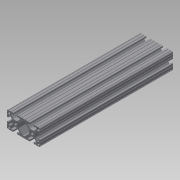
# Autodesk Inventor part: 1530-LITE
Saved by Autodesk Inventor 2013 (Build 170138000, 138)
## iProperties
Created: 2014-04-23
Part Number: 1530-LITE
Material: Generic
Document SubType Name: Modeling
Density: 1 g/cm^3
Vendor: 80/20 Inc.
Engineer: Ross Bowman
Designer: Ross Bowman
Catalog Web Link: 8020.net
Company: 80/20 Inc.
Author: Ross Bowman
Keywords: 80/20 , 8020 , T-Slot , Extrusion
Material: 6105-T5 Aluminum
Autodesk Inventor part; units mm, degrees
ref_plane "YZ Plane" through (0, 0, 0) normal (1, 0, 0) x (0, 1, 0)
ref_plane "XZ Plane" through (0, 0, 0) normal (0, 1, 0) x (-1, 0, 0)
ref_plane "XY Plane" through (0, 0, 0) normal (0, 0, 1) x (1, 0, 0)
sketch "Sketch1" plane through (0, 0, 0) normal (0, 0, 1) x (1, 0, 0)
  arc A0 (-31.2928, -17.2466) -> (-30.9118, -16.8656) centre (-31.2928, -16.8656) ccw
  line L0 (-33.5026, -17.2466) -> (-31.2928, -17.2466)
  arc A1 (-36.2966, -14.4526) -> (-33.5026, -17.2466) centre (-33.5026, -14.4526) ccw
  line L1 (-36.2966, -12.2428) -> (-36.2966, -14.4526)
  arc A2 (-35.9156, -11.8618) -> (-36.2966, -12.2428) centre (-35.9156, -12.2428) ccw
  line L2 (-31.2928, -11.8618) -> (-35.9156, -11.8618)
  arc A3 (-30.9118, -12.2428) -> (-31.2928, -11.8618) centre (-31.2928, -12.2428) ccw
  line L3 (-30.9118, -16.8656) -> (-30.9118, -12.2428)
  arc A4 (2.0655, 14.8293) -> (-2.0655, 14.8293) centre (0, 12.7638) ccw
  line L4 (10.9278, 5.9669) -> (2.0655, 14.8293)
  arc A5 (12.319, 2.6083) -> (10.9278, 5.9669) centre (7.5692, 2.6083) ccw
  line L5 (12.319, -2.6083) -> (12.319, 2.6083)
  arc A6 (10.9278, -5.9669) -> (12.319, -2.6083) centre (7.5692, -2.6083) ccw
  line L6 (2.0655, -14.8293) -> (10.9278, -5.9669)
  arc A7 (-2.0655, -14.8293) -> (2.0655, -14.8293) centre (0, -12.7638) ccw
  line L7 (-10.9278, -5.9669) -> (-2.0655, -14.8293)
  arc A8 (-12.319, -2.6083) -> (-10.9278, -5.9669) centre (-7.5692, -2.6083) ccw
  line L8 (-12.319, 2.6083) -> (-12.319, -2.6083)
  arc A9 (-10.9278, 5.9669) -> (-12.319, 2.6083) centre (-7.5692, 2.6083) ccw
  line L9 (-2.0655, 14.8293) -> (-10.9278, 5.9669)
  circle A10 centre (19.05, 0) radius 3.3274
  arc A11 (30.9118, -16.8656) -> (31.2928, -17.2466) centre (31.2928, -16.8656) ccw
  line L10 (30.9118, -12.2428) -> (30.9118, -16.8656)
  arc A12 (31.2928, -11.8618) -> (30.9118, -12.2428) centre (31.2928, -12.2428) ccw
  line L11 (35.9156, -11.8618) -> (31.2928, -11.8618)
  arc A13 (36.2966, -12.2428) -> (35.9156, -11.8618) centre (35.9156, -12.2428) ccw
  line L12 (36.2966, -14.4526) -> (36.2966, -12.2428)
  arc A14 (33.5026, -17.2466) -> (36.2966, -14.4526) centre (33.5026, -14.4526) ccw
  line L13 (31.2928, -17.2466) -> (33.5026, -17.2466)
  arc A15 (31.2928, 17.2466) -> (30.9118, 16.8656) centre (31.2928, 16.8656) ccw
  line L14 (33.5026, 17.2466) -> (31.2928, 17.2466)
  arc A16 (36.2966, 14.4526) -> (33.5026, 17.2466) centre (33.5026, 14.4526) ccw
  line L15 (36.2966, 12.2428) -> (36.2966, 14.4526)
  arc A17 (35.9156, 11.8618) -> (36.2966, 12.2428) centre (35.9156, 12.2428) ccw
  line L16 (31.2928, 11.8618) -> (35.9156, 11.8618)
  arc A18 (30.9118, 12.2428) -> (31.2928, 11.8618) centre (31.2928, 12.2428) ccw
  line L17 (30.9118, 16.8656) -> (30.9118, 12.2428)
  circle A19 centre (-19.05, 0) radius 3.3274
  arc A20 (-30.9118, 16.8656) -> (-31.2928, 17.2466) centre (-31.2928, 16.8656) ccw
  line L18 (-30.9118, 12.2428) -> (-30.9118, 16.8656)
  arc A21 (-31.2928, 11.8618) -> (-30.9118, 12.2428) centre (-31.2928, 12.2428) ccw
  line L19 (-35.9156, 11.8618) -> (-31.2928, 11.8618)
  arc A22 (-36.2966, 12.2428) -> (-35.9156, 11.8618) centre (-35.9156, 12.2428) ccw
  line L20 (-36.2966, 14.4526) -> (-36.2966, 12.2428)
  arc A23 (-33.5026, 17.2466) -> (-36.2966, 14.4526) centre (-33.5026, 14.4526) ccw
  line L21 (-31.2928, 17.2466) -> (-33.5026, 17.2466)
  arc A24 (-3.2004, -19.05) -> (-4.7244, -19.05) centre (-3.9624, -19.05) ccw
  line L22 (-3.2004, -19.05) -> (3.2004, -19.05)
  arc A25 (4.7244, -19.05) -> (3.2004, -19.05) centre (3.9624, -19.05) ccw
  line L23 (4.7244, -19.05) -> (9.5504, -19.05)
  arc A26 (11.0744, -19.05) -> (9.5504, -19.05) centre (10.3124, -19.05) ccw
  line L24 (11.0744, -19.05) -> (13.4112, -19.05)
  arc A27 (13.4112, -19.05) -> (14.986, -17.4752) centre (13.4112, -17.4752) ccw
  line L25 (14.986, -17.4752) -> (14.986, -16.5608)
  arc A28 (14.986, -16.5608) -> (13.4112, -14.986) centre (13.4112, -16.5608) ccw
  line L26 (13.4112, -14.986) -> (12.573, -14.986)
  arc A29 (12.573, -14.986) -> (12.192, -15.367) centre (12.573, -15.367) ccw
  line L27 (12.192, -15.367) -> (12.192, -15.4432)
  arc A30 (11.811, -15.8242) -> (12.192, -15.4432) centre (11.811, -15.4432) ccw
  line L28 (11.811, -15.8242) -> (10.033, -15.8242)
  arc A31 (8.763, -14.5542) -> (10.033, -15.8242) centre (10.033, -14.5542) ccw
  line L29 (8.763, -14.5542) -> (8.763, -12.9683)
  arc A32 (9.135, -12.0703) -> (8.763, -12.9683) centre (10.033, -12.9683) ccw
  line L30 (9.135, -12.0703) -> (13.0831, -8.1222)
  arc A33 (16.4417, -6.731) -> (13.0831, -8.1222) centre (16.4417, -11.4808) ccw
  line L31 (16.4417, -6.731) -> (21.6583, -6.731)
  arc A34 (25.0169, -8.1222) -> (21.6583, -6.731) centre (21.6583, -11.4808) ccw
  line L32 (25.0169, -8.1222) -> (28.965, -12.0703)
  arc A35 (29.337, -12.9683) -> (28.965, -12.0703) centre (28.067, -12.9683) ccw
  line L33 (29.337, -12.9683) -> (29.337, -14.5542)
  arc A36 (28.067, -15.8242) -> (29.337, -14.5542) centre (28.067, -14.5542) ccw
  line L34 (28.067, -15.8242) -> (26.289, -15.8242)
  arc A37 (25.908, -15.4432) -> (26.289, -15.8242) centre (26.289, -15.4432) ccw
  line L35 (25.908, -15.4432) -> (25.908, -15.367)
  arc A38 (25.908, -15.367) -> (25.527, -14.986) centre (25.527, -15.367) ccw
  line L36 (25.527, -14.986) -> (24.6888, -14.986)
  arc A39 (24.6888, -14.986) -> (23.114, -16.5608) centre (24.6888, -16.5608) ccw
  line L37 (23.114, -16.5608) -> (23.114, -17.4752)
  arc A40 (23.114, -17.4752) -> (24.6888, -19.05) centre (24.6888, -17.4752) ccw
  line L38 (24.6888, -19.05) -> (27.0256, -19.05)
  arc A41 (28.5496, -19.05) -> (27.0256, -19.05) centre (27.7876, -19.05) ccw
  line L39 (28.5496, -19.05) -> (33.3756, -19.05)
  arc A42 (34.8996, -19.05) -> (33.3756, -19.05) centre (34.1376, -19.05) ccw
  line L40 (34.8996, -19.05) -> (34.925, -19.05)
  arc A43 (34.925, -19.05) -> (38.1, -15.875) centre (34.925, -15.875) ccw
  line L41 (38.1, -15.875) -> (38.1, -15.8496)
  arc A44 (38.1, -14.3256) -> (38.1, -15.8496) centre (38.1, -15.0876) ccw
  line L42 (38.1, -14.3256) -> (38.1, -9.4996)
  arc A45 (38.1, -7.9756) -> (38.1, -9.4996) centre (38.1, -8.7376) ccw
  line L43 (38.1, -7.9756) -> (38.1, -5.6388)
  arc A46 (38.1, -5.6388) -> (36.5252, -4.064) centre (36.5252, -5.6388) ccw
  line L44 (36.5252, -4.064) -> (35.6108, -4.064)
  arc A47 (35.6108, -4.064) -> (34.036, -5.6388) centre (35.6108, -5.6388) ccw
  line L45 (34.036, -5.6388) -> (34.036, -6.477)
  arc A48 (34.036, -6.477) -> (34.417, -6.858) centre (34.417, -6.477) ccw
  line L46 (34.417, -6.858) -> (34.4932, -6.858)
  arc A49 (34.8742, -7.239) -> (34.4932, -6.858) centre (34.4932, -7.239) ccw
  line L47 (34.8742, -7.239) -> (34.8742, -9.017)
  arc A50 (33.6042, -10.287) -> (34.8742, -9.017) centre (33.6042, -9.017) ccw
  line L48 (33.6042, -10.287) -> (32.0183, -10.287)
  arc A51 (31.1203, -9.915) -> (32.0183, -10.287) centre (32.0183, -9.017) ccw
  line L49 (31.1203, -9.915) -> (27.1722, -5.9669)
  arc A52 (25.781, -2.6083) -> (27.1722, -5.9669) centre (30.5308, -2.6083) ccw
  line L50 (25.781, -2.6083) -> (25.781, 2.6083)
  arc A53 (27.1722, 5.9669) -> (25.781, 2.6083) centre (30.5308, 2.6083) ccw
  line L51 (27.1722, 5.9669) -> (31.1203, 9.915)
  arc A54 (32.0183, 10.287) -> (31.1203, 9.915) centre (32.0183, 9.017) ccw
  line L52 (32.0183, 10.287) -> (33.6042, 10.287)
  arc A55 (34.8742, 9.017) -> (33.6042, 10.287) centre (33.6042, 9.017) ccw
  line L53 (34.8742, 9.017) -> (34.8742, 7.239)
  arc A56 (34.4932, 6.858) -> (34.8742, 7.239) centre (34.4932, 7.239) ccw
  line L54 (34.4932, 6.858) -> (34.417, 6.858)
  arc A57 (34.417, 6.858) -> (34.036, 6.477) centre (34.417, 6.477) ccw
  line L55 (34.036, 6.477) -> (34.036, 5.6388)
  arc A58 (34.036, 5.6388) -> (35.6108, 4.064) centre (35.6108, 5.6388) ccw
  line L56 (35.6108, 4.064) -> (36.5252, 4.064)
  arc A59 (36.5252, 4.064) -> (38.1, 5.6388) centre (36.5252, 5.6388) ccw
  line L57 (38.1, 5.6388) -> (38.1, 7.9756)
  arc A60 (38.1, 9.4996) -> (38.1, 7.9756) centre (38.1, 8.7376) ccw
  line L58 (38.1, 9.4996) -> (38.1, 14.3256)
  arc A61 (38.1, 15.8496) -> (38.1, 14.3256) centre (38.1, 15.0876) ccw
  line L59 (38.1, 15.8496) -> (38.1, 15.875)
  arc A62 (38.1, 15.875) -> (34.925, 19.05) centre (34.925, 15.875) ccw
  line L60 (34.925, 19.05) -> (34.8996, 19.05)
  arc A63 (33.3756, 19.05) -> (34.8996, 19.05) centre (34.1376, 19.05) ccw
  line L61 (33.3756, 19.05) -> (28.5496, 19.05)
  arc A64 (27.0256, 19.05) -> (28.5496, 19.05) centre (27.7876, 19.05) ccw
  line L62 (27.0256, 19.05) -> (24.6888, 19.05)
  arc A65 (24.6888, 19.05) -> (23.114, 17.4752) centre (24.6888, 17.4752) ccw
  line L63 (23.114, 17.4752) -> (23.114, 16.5608)
  arc A66 (23.114, 16.5608) -> (24.6888, 14.986) centre (24.6888, 16.5608) ccw
  line L64 (24.6888, 14.986) -> (25.527, 14.986)
  arc A67 (25.527, 14.986) -> (25.908, 15.367) centre (25.527, 15.367) ccw
  line L65 (25.908, 15.367) -> (25.908, 15.4432)
  arc A68 (26.289, 15.8242) -> (25.908, 15.4432) centre (26.289, 15.4432) ccw
  line L66 (26.289, 15.8242) -> (28.067, 15.8242)
  arc A69 (29.337, 14.5542) -> (28.067, 15.8242) centre (28.067, 14.5542) ccw
  line L67 (29.337, 14.5542) -> (29.337, 12.9683)
  arc A70 (28.965, 12.0703) -> (29.337, 12.9683) centre (28.067, 12.9683) ccw
  line L68 (28.965, 12.0703) -> (25.0169, 8.1222)
  arc A71 (21.6583, 6.731) -> (25.0169, 8.1222) centre (21.6583, 11.4808) ccw
  line L69 (21.6583, 6.731) -> (16.4417, 6.731)
  arc A72 (13.0831, 8.1222) -> (16.4417, 6.731) centre (16.4417, 11.4808) ccw
  line L70 (13.0831, 8.1222) -> (9.135, 12.0703)
  arc A73 (8.763, 12.9683) -> (9.135, 12.0703) centre (10.033, 12.9683) ccw
  line L71 (8.763, 12.9683) -> (8.763, 14.5542)
  arc A74 (10.033, 15.8242) -> (8.763, 14.5542) centre (10.033, 14.5542) ccw
  line L72 (10.033, 15.8242) -> (11.811, 15.8242)
  arc A75 (12.192, 15.4432) -> (11.811, 15.8242) centre (11.811, 15.4432) ccw
  line L73 (12.192, 15.4432) -> (12.192, 15.367)
  arc A76 (12.192, 15.367) -> (12.573, 14.986) centre (12.573, 15.367) ccw
  line L74 (12.573, 14.986) -> (13.4112, 14.986)
  arc A77 (13.4112, 14.986) -> (14.986, 16.5608) centre (13.4112, 16.5608) ccw
  line L75 (14.986, 16.5608) -> (14.986, 17.4752)
  arc A78 (14.986, 17.4752) -> (13.4112, 19.05) centre (13.4112, 17.4752) ccw
  line L76 (13.4112, 19.05) -> (11.0744, 19.05)
  arc A79 (9.5504, 19.05) -> (11.0744, 19.05) centre (10.3124, 19.05) ccw
  line L77 (9.5504, 19.05) -> (4.7244, 19.05)
  arc A80 (3.2004, 19.05) -> (4.7244, 19.05) centre (3.9624, 19.05) ccw
  line L78 (3.2004, 19.05) -> (-3.2004, 19.05)
  arc A81 (-4.7244, 19.05) -> (-3.2004, 19.05) centre (-3.9624, 19.05) ccw
  line L79 (-4.7244, 19.05) -> (-9.5504, 19.05)
  arc A82 (-11.0744, 19.05) -> (-9.5504, 19.05) centre (-10.3124, 19.05) ccw
  line L80 (-11.0744, 19.05) -> (-13.4112, 19.05)
  arc A83 (-13.4112, 19.05) -> (-14.986, 17.4752) centre (-13.4112, 17.4752) ccw
  line L81 (-14.986, 17.4752) -> (-14.986, 16.5608)
  arc A84 (-14.986, 16.5608) -> (-13.4112, 14.986) centre (-13.4112, 16.5608) ccw
  line L82 (-13.4112, 14.986) -> (-12.573, 14.986)
  arc A85 (-12.573, 14.986) -> (-12.192, 15.367) centre (-12.573, 15.367) ccw
  line L83 (-12.192, 15.367) -> (-12.192, 15.4432)
  arc A86 (-11.811, 15.8242) -> (-12.192, 15.4432) centre (-11.811, 15.4432) ccw
  line L84 (-11.811, 15.8242) -> (-10.033, 15.8242)
  arc A87 (-8.763, 14.5542) -> (-10.033, 15.8242) centre (-10.033, 14.5542) ccw
  line L85 (-8.763, 14.5542) -> (-8.763, 12.9683)
  arc A88 (-9.135, 12.0703) -> (-8.763, 12.9683) centre (-10.033, 12.9683) ccw
  line L86 (-9.135, 12.0703) -> (-13.0831, 8.1222)
  arc A89 (-16.4417, 6.731) -> (-13.0831, 8.1222) centre (-16.4417, 11.4808) ccw
  line L87 (-16.4417, 6.731) -> (-21.6583, 6.731)
  arc A90 (-25.0169, 8.1222) -> (-21.6583, 6.731) centre (-21.6583, 11.4808) ccw
  line L88 (-25.0169, 8.1222) -> (-28.965, 12.0703)
  arc A91 (-29.337, 12.9683) -> (-28.965, 12.0703) centre (-28.067, 12.9683) ccw
  line L89 (-29.337, 12.9683) -> (-29.337, 14.5542)
  arc A92 (-28.067, 15.8242) -> (-29.337, 14.5542) centre (-28.067, 14.5542) ccw
  line L90 (-28.067, 15.8242) -> (-26.289, 15.8242)
  arc A93 (-25.908, 15.4432) -> (-26.289, 15.8242) centre (-26.289, 15.4432) ccw
  line L91 (-25.908, 15.4432) -> (-25.908, 15.367)
  arc A94 (-25.908, 15.367) -> (-25.527, 14.986) centre (-25.527, 15.367) ccw
  line L92 (-25.527, 14.986) -> (-24.6888, 14.986)
  arc A95 (-24.6888, 14.986) -> (-23.114, 16.5608) centre (-24.6888, 16.5608) ccw
  line L93 (-23.114, 16.5608) -> (-23.114, 17.4752)
  arc A96 (-23.114, 17.4752) -> (-24.6888, 19.05) centre (-24.6888, 17.4752) ccw
  line L94 (-24.6888, 19.05) -> (-27.0256, 19.05)
  arc A97 (-28.5496, 19.05) -> (-27.0256, 19.05) centre (-27.7876, 19.05) ccw
  line L95 (-28.5496, 19.05) -> (-33.3756, 19.05)
  arc A98 (-34.8996, 19.05) -> (-33.3756, 19.05) centre (-34.1376, 19.05) ccw
  line L96 (-34.8996, 19.05) -> (-34.925, 19.05)
  arc A99 (-34.925, 19.05) -> (-38.1, 15.875) centre (-34.925, 15.875) ccw
  line L97 (-38.1, 15.875) -> (-38.1, 15.8496)
  arc A100 (-38.1, 14.3256) -> (-38.1, 15.8496) centre (-38.1, 15.0876) ccw
  line L98 (-38.1, 14.3256) -> (-38.1, 9.4996)
  arc A101 (-38.1, 7.9756) -> (-38.1, 9.4996) centre (-38.1, 8.7376) ccw
  line L99 (-38.1, 7.9756) -> (-38.1, 5.6388)
  arc A102 (-38.1, 5.6388) -> (-36.5252, 4.064) centre (-36.5252, 5.6388) ccw
  line L100 (-36.5252, 4.064) -> (-35.6108, 4.064)
  arc A103 (-35.6108, 4.064) -> (-34.036, 5.6388) centre (-35.6108, 5.6388) ccw
  line L101 (-34.036, 5.6388) -> (-34.036, 6.477)
  arc A104 (-34.036, 6.477) -> (-34.417, 6.858) centre (-34.417, 6.477) ccw
  line L102 (-34.417, 6.858) -> (-34.4932, 6.858)
  arc A105 (-34.8742, 7.239) -> (-34.4932, 6.858) centre (-34.4932, 7.239) ccw
  line L103 (-34.8742, 7.239) -> (-34.8742, 9.017)
  arc A106 (-33.6042, 10.287) -> (-34.8742, 9.017) centre (-33.6042, 9.017) ccw
  line L104 (-33.6042, 10.287) -> (-32.0183, 10.287)
  arc A107 (-31.1203, 9.915) -> (-32.0183, 10.287) centre (-32.0183, 9.017) ccw
  line L105 (-31.1203, 9.915) -> (-27.1722, 5.9669)
  arc A108 (-25.781, 2.6083) -> (-27.1722, 5.9669) centre (-30.5308, 2.6083) ccw
  line L106 (-25.781, 2.6083) -> (-25.781, -2.6083)
  arc A109 (-27.1722, -5.9669) -> (-25.781, -2.6083) centre (-30.5308, -2.6083) ccw
  line L107 (-27.1722, -5.9669) -> (-31.1203, -9.915)
  arc A110 (-32.0183, -10.287) -> (-31.1203, -9.915) centre (-32.0183, -9.017) ccw
  line L108 (-32.0183, -10.287) -> (-33.6042, -10.287)
  arc A111 (-34.8742, -9.017) -> (-33.6042, -10.287) centre (-33.6042, -9.017) ccw
  line L109 (-34.8742, -9.017) -> (-34.8742, -7.239)
  arc A112 (-34.4932, -6.858) -> (-34.8742, -7.239) centre (-34.4932, -7.239) ccw
  line L110 (-34.4932, -6.858) -> (-34.417, -6.858)
  arc A113 (-34.417, -6.858) -> (-34.036, -6.477) centre (-34.417, -6.477) ccw
  line L111 (-34.036, -6.477) -> (-34.036, -5.6388)
  arc A114 (-34.036, -5.6388) -> (-35.6108, -4.064) centre (-35.6108, -5.6388) ccw
  line L112 (-35.6108, -4.064) -> (-36.5252, -4.064)
  arc A115 (-36.5252, -4.064) -> (-38.1, -5.6388) centre (-36.5252, -5.6388) ccw
  line L113 (-38.1, -5.6388) -> (-38.1, -7.9756)
  arc A116 (-38.1, -9.4996) -> (-38.1, -7.9756) centre (-38.1, -8.7376) ccw
  line L114 (-38.1, -9.4996) -> (-38.1, -14.3256)
  arc A117 (-38.1, -15.8496) -> (-38.1, -14.3256) centre (-38.1, -15.0876) ccw
  line L115 (-38.1, -15.8496) -> (-38.1, -15.875)
  arc A118 (-38.1, -15.875) -> (-34.925, -19.05) centre (-34.925, -15.875) ccw
  line L116 (-34.925, -19.05) -> (-34.8996, -19.05)
  arc A119 (-33.3756, -19.05) -> (-34.8996, -19.05) centre (-34.1376, -19.05) ccw
  line L117 (-33.3756, -19.05) -> (-28.5496, -19.05)
  arc A120 (-27.0256, -19.05) -> (-28.5496, -19.05) centre (-27.7876, -19.05) ccw
  line L118 (-27.0256, -19.05) -> (-24.6888, -19.05)
  arc A121 (-24.6888, -19.05) -> (-23.114, -17.4752) centre (-24.6888, -17.4752) ccw
  line L119 (-23.114, -17.4752) -> (-23.114, -16.5608)
  arc A122 (-23.114, -16.5608) -> (-24.6888, -14.986) centre (-24.6888, -16.5608) ccw
  line L120 (-24.6888, -14.986) -> (-25.527, -14.986)
  arc A123 (-25.527, -14.986) -> (-25.908, -15.367) centre (-25.527, -15.367) ccw
  line L121 (-25.908, -15.367) -> (-25.908, -15.4432)
  arc A124 (-26.289, -15.8242) -> (-25.908, -15.4432) centre (-26.289, -15.4432) ccw
  line L122 (-26.289, -15.8242) -> (-28.067, -15.8242)
  arc A125 (-29.337, -14.5542) -> (-28.067, -15.8242) centre (-28.067, -14.5542) ccw
  line L123 (-29.337, -14.5542) -> (-29.337, -12.9683)
  arc A126 (-28.965, -12.0703) -> (-29.337, -12.9683) centre (-28.067, -12.9683) ccw
  line L124 (-28.965, -12.0703) -> (-25.0169, -8.1222)
  arc A127 (-21.6583, -6.731) -> (-25.0169, -8.1222) centre (-21.6583, -11.4808) ccw
  line L125 (-21.6583, -6.731) -> (-16.4417, -6.731)
  arc A128 (-13.0831, -8.1222) -> (-16.4417, -6.731) centre (-16.4417, -11.4808) ccw
  line L126 (-13.0831, -8.1222) -> (-9.135, -12.0703)
  arc A129 (-8.763, -12.9683) -> (-9.135, -12.0703) centre (-10.033, -12.9683) ccw
  line L127 (-8.763, -12.9683) -> (-8.763, -14.5542)
  arc A130 (-10.033, -15.8242) -> (-8.763, -14.5542) centre (-10.033, -14.5542) ccw
  line L128 (-10.033, -15.8242) -> (-11.811, -15.8242)
  arc A131 (-12.192, -15.4432) -> (-11.811, -15.8242) centre (-11.811, -15.4432) ccw
  line L129 (-12.192, -15.4432) -> (-12.192, -15.367)
  arc A132 (-12.192, -15.367) -> (-12.573, -14.986) centre (-12.573, -15.367) ccw
  line L130 (-12.573, -14.986) -> (-13.4112, -14.986)
  arc A133 (-13.4112, -14.986) -> (-14.986, -16.5608) centre (-13.4112, -16.5608) ccw
  line L131 (-14.986, -16.5608) -> (-14.986, -17.4752)
  arc A134 (-14.986, -17.4752) -> (-13.4112, -19.05) centre (-13.4112, -17.4752) ccw
  line L132 (-13.4112, -19.05) -> (-11.0744, -19.05)
  arc A135 (-9.5504, -19.05) -> (-11.0744, -19.05) centre (-10.3124, -19.05) ccw
  line L133 (-9.5504, -19.05) -> (-4.7244, -19.05)
  point P0 (0, 0)
  constraints: 268 end point, 268 point on circle, 136 centre point
extrude "Extrusion1" add sketch "Sketch1" against normal blind 304.8
body "Solid1"
